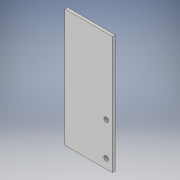
# Autodesk Inventor part: BatteryBracketLeft
Saved by Autodesk Inventor 2019.3 (Build 233278000, 278)
## iProperties
Created: 2019-01-26
Part Number: BatteryBracketLeft
Material: Generic
Document SubType Name: Modeling
Designer: mark
Density: 1 g/cm^3
Appearance: Default
Author: mark
Autodesk Inventor part; units mm, degrees
ref_plane "YZ Plane" through (0, 0, 0) normal (1, 0, 0) x (0, 1, 0)
ref_plane "XZ Plane" through (0, 0, 0) normal (0, 1, 0) x (-1, 0, 0)
ref_plane "XY Plane" through (0, 0, 0) normal (0, 0, 1) x (1, 0, 0)
sketch "Sketch1" plane through (0, 0, 0) normal (0, 0, 1) x (1, 0, 0)
  line L0 (50.75, 0) -> (50.75, 125.8)
  line L1 (50.75, 125.8) -> (0, 125.8)
  line L2 (0, 125.8) -> (0, 0)
  circle A0 centre (44.25, 10) radius 2.5
  circle A1 centre (44.25, 45.7) radius 2.5
  line L3 (0, 0) -> (50.75, 0)
  dimension "d0" = 50.75
  dimension "d1" = 125.8
  dimension "d2" = 5
  dimension "d3" = 5
  dimension "d14" = 10
  dimension "d15" = 35.7
  dimension "d16" = 6.5
  dimension "d17" = 6.5
  constraints: 8 end point, 3 perpendicular, 2 centre point, 1 horizontal
  measures "d0" distance of L1.end L0.end
  measures "d1" distance of L0.end L0.start
  measures "d2" diameter of A0
  measures "d3" diameter of A1
  measures "d14" distance from line of L3 A0.centre
  measures "d15" distance of A1.centre A0.centre
  measures "d16" distance from line of L0 A1.centre
  measures "d17" distance from line of A0.centre L0
extrude "Extrusion1" add sketch "Sketch1" along normal blind 3.1
body "Solid1"
